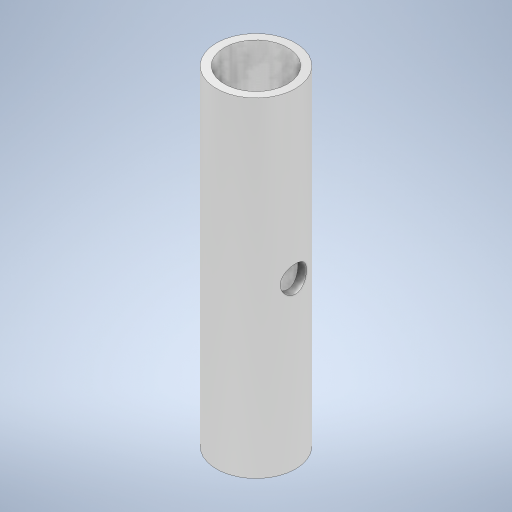
# Autodesk Inventor part: InsertTube6OD0.6W25L
Saved by Autodesk Inventor 2024 (Build 280153000, 153)
## iProperties
Created: 2023-09-24
Part Number: InsertTube6OD0.6W25L
Material: Stainless Steel AISI 304
Document SubType Name: Modeling
Designer: schanen
Density: 8 g/cm^3
Appearance: Chrome - Satin
Author: schanen
Autodesk Inventor part; units mm, degrees
ref_plane "XZ Plane" through (0, 0, 0) normal (0, 1, 0) x (-1, 0, 0)
sketch "Sketch1" plane through (0, 0, 0) normal (0, 0, 1) x (1, 0, 0)
  line L0 (-2.4, 0) -> (-3, 0)
  line L1 (-3, 0) -> (-3, 25)
  line L2 (-3, 25) -> (-2.4, 25)
  line L3 (-2.4, 25) -> (-2.4, 0)
  line L4 (0, -5) -> (0, 30) projected
  point P0 (0, 0)
  dimension "d0" = 3
  dimension "d1" = 0.6
  dimension "d2" = 25
  constraints: 8 end point, 2 parallel, 1 horizontal, 1 perpendicular
  measures "d0" distance from line of point (0, 0) L1
  measures "d1" distance between parallel lines of L1 L3
  measures "d2" distance of L0.end L1.end
revolve "Revolution1" add sketch "Sketch1" angle 360 about axis through (0, -10, 0) along (0, 1, 0)
ref_plane "Work Plane1" through (0, 12.5, 0) normal (0, 1, 0) x (1, 0, 0)
ref_plane "Work Plane2" through (0, 0, 0) normal (1, 0, 0) x (0, 1, 0)
sketch "Sketch2" plane through (0, 0, 0) normal (1, 0, 0) x (0, 1, 0)
  line L0 (12.5, 4.2) -> (12.5, -4.2) projected
  line L1 (-10, 0) -> (60, 0) projected
  point P0 (0, 0)
  point P1 (12.5, 0)
  constraints: 1 midpoint, 1 point on line
hole "Hole1" at (0, 12.5, 0) direction (-1, 0, 0) diameter 2 end through all both
body "Solid1"
